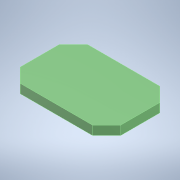
# Autodesk Inventor part: FactionSpecial_Council_ControlMarker_Single
Saved by Autodesk Inventor 2021 (Build 250183000, 183)
## iProperties
Created: 2023-03-16
Part Number: FactionSpecial_Council_ControlMarker_Single
Material: ABS Plastic
Document SubType Name: Modeling
Designer: Bradley
Density: 1.06 g/cm^3
Appearance: Smooth - Dark Forest Green
CouncilCMWidth: 21.200 mm
CouncilCMHeight: 14.200 mm
CouncilCMChamfer: 3.000 mm
Author: Bradley
Autodesk Inventor part; units mm, degrees
ref_plane "YZ Plane" through (0, 0, 0) normal (1, 0, 0) x (0, 1, 0)
ref_plane "XZ Plane" through (0, 0, 0) normal (0, 1, 0) x (-1, 0, 0)
ref_plane "XY Plane" through (0, 0, 0) normal (0, 0, 1) x (1, 0, 0)
sketch "Sketch1" plane through (0, 0, 0) normal (0, 1, 0) x (-1, 0, 0)
  line L0 (7.6, 7.1) -> (-7.6, 7.1)
  line L1 (-10.6, 4.1) -> (-10.6, -4.1)
  line L2 (-7.6, -7.1) -> (7.6, -7.1)
  line L3 (10.6, -4.1) -> (10.6, 4.1)
  line L4 (10.6, 7.1) -> (-10.6, -7.1) construction
  line L5 (-10.6, 7.1) -> (10.6, -7.1) construction
  line L6 (7.6, -7.1) -> (10.6, -4.1)
  line L7 (10.6, 4.1) -> (7.6, 7.1)
  line L8 (-7.6, 7.1) -> (-10.6, 4.1)
  line L9 (-10.6, -4.1) -> (-7.6, -7.1)
  point P0 (0, 0)
  dimension "d0" = 21.2
  dimension "d1" = 14.2
  dimension "d2" = 3
  dimension "d3" = 3
  dimension "d12" = 20.7889
  constraints: 20 end point, 8 point on line, 7 perpendicular, 2 midpoint, 2 parallel, 1 horizontal
  measures "d0" distance of L5.end L4.end
  measures "d1" distance of L4.end L5.start
  measures "d2" distance of L2.end L5.end
  measures "d3" distance of L3.start L5.end
  measures "d12" distance between parallel lines of L8 L6
extrude "Extrusion1" add sketch "Sketch1" along normal mid plane 1.9
equation "\"d0\" = CouncilCMWidth"
equation "\"d1\" = CouncilCMHeight"
equation "\"d2\" = CouncilCMChamfer"
equation "\"d3\" = d2"
equation "\"CouncilCMWidth\" = 21.2"
equation "\"CouncilCMHeight\" = 14.2"
equation "\"CouncilCMChamfer\" = 3"
body "Solid1"
